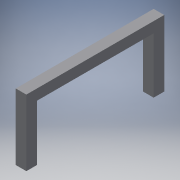
# Autodesk Inventor part: Part100
Saved by Autodesk Inventor 2016 (Build 200138000, 138)
## iProperties
Created: 2016-09-06
Part Number: Part100
Material: Aluminum 6061
Document SubType Name: Modeling
Designer: gus
Density: 2.7 g/cm^3
Appearance: Aluminum - Flat
Author: gus
Autodesk Inventor part; units mm, degrees
ref_plane "YZ Plane" through (0, 0, 0) normal (1, 0, 0) x (0, 1, 0)
ref_plane "XZ Plane" through (0, 0, 0) normal (0, 1, 0) x (-1, 0, 0)
ref_plane "XY Plane" through (0, 0, 0) normal (0, 0, 1) x (1, 0, 0)
sketch "Sketch1" plane through (0, 0, 0) normal (1, 0, 0) x (0, 1, 0)
  line L0 (0, 0) -> (0, 25.4)
  line L1 (0, 25.4) -> (133.35, 25.4)
  line L2 (133.35, 25.4) -> (133.35, 304.8)
  line L3 (133.35, 304.8) -> (0, 304.8)
  line L4 (0, 304.8) -> (0, 330.2)
  line L5 (0, 330.2) -> (158.75, 330.2)
  line L6 (158.75, 330.2) -> (158.75, 0)
  line L7 (158.75, 0) -> (0, 0)
  dimension "d0" = 158.75
  dimension "d1" = 25.4
  dimension "d2" = 330.2
  dimension "d3" = 25.4
  dimension "d4" = 25.4
  constraints: 16 end point, 6 perpendicular, 2 point on line, 1 vertical
  measures "d0" distance of L6.end L0.start
  measures "d1" distance between parallel lines of L6 L2
  measures "d2" distance of L5.end L6.end
  measures "d3" distance of L3.end L4.end
  measures "d4" distance of L0.start L0.end
extrude "Extrusion1" add sketch "Sketch1" along normal blind 25.4
body "Solid1"
